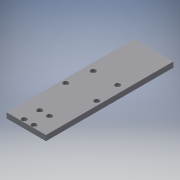
# Autodesk Inventor part: suporte_cabeça_superior
Saved by Autodesk Inventor 2018 (Build 220112000, 112)
## iProperties
Created: 2018-05-17
Part Number: suporte_cabeça_superior
Material: Genérico
Document SubType Name: Modeling
Designer: Usuario
Density: 1 g/cm^3
Appearance: Padrão
Author: Usuario
Autodesk Inventor part; units mm, degrees
ref_plane "YZ Plane" through (0, 0, 0) normal (1, 0, 0) x (0, 1, 0)
ref_plane "XZ Plane" through (0, 0, 0) normal (0, 1, 0) x (-1, 0, 0)
ref_plane "XY Plane" through (0, 0, 0) normal (0, 0, 1) x (1, 0, 0)
sketch "Esboço2" plane through (0, 0, 0) normal (0, 0, 1) x (1, 0, 0)
  line L0 (-1.4393, 191.951) -> (-2.5, 191.951) construction
  line L1 (-2.5, 191.951) -> (-2.5, 190.8903) construction
  line L2 (67.4393, -37.951) -> (68.5, -37.951) construction
  line L3 (68.5, -37.951) -> (68.5, -36.8903) construction
  line L4 (-2.5, 191.951) -> (68.5, 191.951)
  line L5 (68.5, 191.951) -> (68.5, -37.951)
  line L6 (68.5, -37.951) -> (-2.5, -37.951)
  line L7 (-2.5, -37.951) -> (-2.5, 191.951)
  point P0 (0, 0)
  dimension "d14" = 71
  constraints: 16 end point, 3 horizontal, 3 perpendicular, 2 parallel
  measures "d14" distance between parallel lines of L7 L5
extrude "Extrusão2" add sketch "Esboço2" along normal blind 9.5
sketch "Esboço3" plane through (0, 0, 9.5) normal (0, 0, 1) x (1, 0, 0)
  point P0 (0, 0)
  point P1 (41.8302, -5)
  point P2 (24.1698, -5)
  point P3 (41.8302, -33)
  point P4 (24.1698, -33)
  point P5 (54.985, 104.9)
  point P6 (11.015, 104.9)
  point P7 (5, 61.2)
  point P8 (61, 61.2)
hole "Furo1" at (11.015, 104.9, 9.5) at (54.985, 104.9, 9.5) at (5, 61.2, 9.5) at (61, 61.2, 9.5) at (24.1698, -5, 9.5) at (41.8302, -5, 9.5) at (24.1698, -33, 9.5) at (41.8302, -33, 9.5) direction (0, 0, -1) diameter 4 end through all counterbore diameter 9 counterbore depth 5.5
